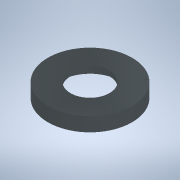
# Autodesk Inventor part: Корпус сальника
Saved by Autodesk Inventor 2021 (Build 250183000, 183)
## iProperties
Created: 2020-11-05
Part Number: Корпус сальника
Material: Чугун, серый
Document SubType Name: Modeling
Designer: Тимоха
Density: 7.15 g/cm^3
Appearance: Чугун серый
Mass: 1505.16 g
Surface Area: 407.904 cm^2
Volume: 210.512 cm^3
Author: Тимоха
Autodesk Inventor part; units mm, degrees
ref_plane "YZ Plane" through (0, 0, 0) normal (1, 0, 0) x (0, 1, 0)
ref_plane "XZ Plane" through (0, 0, 0) normal (0, 1, 0) x (-1, 0, 0)
ref_plane "XY Plane" through (0, 0, 0) normal (0, 0, 1) x (1, 0, 0)
sketch "Эскиз1" plane through (0, 0, 0) normal (0, 0, 1) x (1, 0, 0)
  line L0 (0, 0) -> (0, 20)
  line L1 (69, 0) -> (49, 0)
  line L2 (49, 0) -> (49, 15)
  line L3 (32, 20) -> (32, 15)
  line L4 (32, 15) -> (32, 23)
  line L5 (32, 23) -> (69, 23)
  line L6 (69, 0) -> (69, 23)
  line L7 (32, 15) -> (49, 15)
  line L8 (0, 0) -> (0, 24)
  line L9 (0, 0) -> (0, 30)
  line L10 (0, 30) -> (-75, 30)
  line L11 (-75, 30) -> (-75, 0)
  line L12 (-75, 0) -> (-51, 0)
  line L13 (-51, 0) -> (-51, 15)
  line L14 (-51, 15) -> (-34, 15)
  line L15 (-34, 15) -> (-34, 30)
  dimension "d2" = 20
  dimension "d3" = 15
  dimension "d4" = 32
  dimension "d6" = 8
  dimension "d7" = 17
  dimension "d20" = 30
  dimension "d21" = 75
  dimension "d22" = 24
  dimension "d23" = 15
  dimension "d24" = 17
  constraints: 32 end point, 6 perpendicular, 4 point on line, 2 horizontal, 2 vertical
  measures "d2" distance of L1.start L1.end
  measures "d3" distance of L1.end L2.end
  measures "d4" distance of L0.end L3.start
  measures "d6" distance of L3.end L4.end
  measures "d7" distance of L3.end L2.end
  measures "d20" distance of L0.start L9.end
  measures "d21" distance of L9.end L10.end
  measures "d22" distance of L11.end L12.end
  measures "d23" distance of L12.end L13.end
  measures "d24" distance of L13.end L14.end
revolve "Вращение1" add sketch "Эскиз1" angle 360 about axis through (0, 0, 0) along (0, 1, 0) contours L1 L2 L7 L3 L4 L5 L6
sketch "Эскиз2" plane through (0, 23, 0) normal (0, 1, 0) x (1, 0, 0)
  circle A0 centre (0, 0) radius 32 projected
  circle A1 centre (0, 0) radius 69 projected
  line L0 (0, 0) -> (41.7812, 49.7929)
  line L1 (0, 0) -> (65, 0) construction
  circle A2 centre (41.7812, 49.7929) radius 1.5
  line L2 (0, 0) -> (-32.5, 56.2917)
  line L3 (0, 0) -> (65, 0) construction
  circle A3 centre (-32.5, 56.2917) radius 1.5
  line L4 (0, 0) -> (-11.2871, -64.0125)
  line L5 (0, 0) -> (65, 0) construction
  circle A4 centre (-11.2871, -64.0125) radius 1.5
  dimension "d8" = 65
  dimension "d9" = 50
  dimension "d10" = 3
  dimension "d11" = 65
  dimension "d12" = 120
  dimension "d13" = 3
  dimension "d14" = 65
  dimension "d15" = 100
  dimension "d16" = 3
  constraints: 12 end point, 3 centre point, 3 coincident, 3 equal length, 3 horizontal, 1 point on line
  measures "d8" distance of L0.start L0.end
  measures "d9" angle of L1 L0
  measures "d10" diameter of A2
  measures "d11" distance of L0.start L2.end
  measures "d12" angle of L3 L2
  measures "d13" diameter of A3
  measures "d14" distance of L0.start L4.end
  measures "d15" angle of L4 L5
  measures "d16" diameter of A4
extrude "Выдавливание1" cut sketch "Эскиз2" against normal through all contours A2 | A3 | A4
